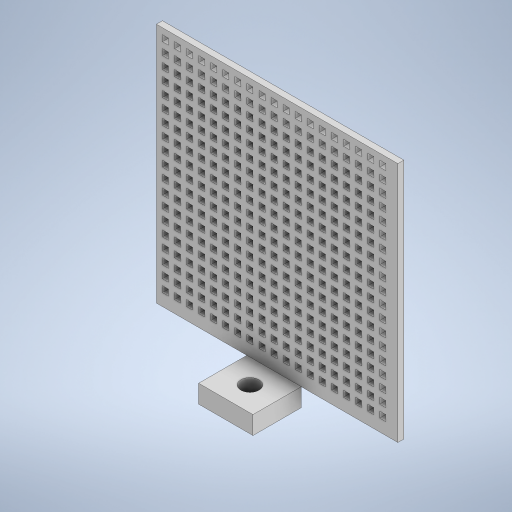
# Autodesk Inventor part: grating20
Saved by Autodesk Inventor 2023 (Build 270158000, 158)
## iProperties
Created: 2022-05-17
Part Number: grating20
Material: Generisch
Document SubType Name: Modeling
Designer: Tim Stechel
Density: 1 g/cm^3
Appearance: Vorgabe
Author: Tim Stechel
Autodesk Inventor part; units mm, degrees
ref_plane "YZ Plane" through (0, 0, 0) normal (1, 0, 0) x (0, 1, 0)
ref_plane "XZ Plane" through (0, 0, 0) normal (0, 1, 0) x (-1, 0, 0)
ref_plane "XY Plane" through (0, 0, 0) normal (0, 0, 1) x (1, 0, 0)
sketch "Skizze1" plane through (0, 0, 0) normal (0, 0, 1) x (1, 0, 0)
  line L0 (-20, 20) -> (20, 20)
  line L1 (20, 20) -> (20, -20)
  line L2 (20, -20) -> (-20, -20)
  line L3 (-20, -20) -> (-20, 20)
  line L4 (0, 2.5115) -> (0, -3.4037)
  line L5 (3.1615, 0) -> (-2.0751, 0)
  line L6 (-20, 20) -> (-19.6762, 20)
  line L7 (-20, 20) -> (-19.6762, 20)
  line L8 (-20, 20) -> (-19, 20)
  line L9 (-19, 20) -> (-18, 20)
  line L10 (-20, 20) -> (-19, 20)
  line L11 (-20, 20) -> (-19, 20)
  line L12 (-20, 20) -> (-19, 20)
  line L13 (-19, 20) -> (-18, 20)
  line L14 (-19, 20) -> (-19, -20)
  line L15 (-18, 20) -> (-18, -20)
  line L16 (-18, 20) -> (-17, 20)
  line L17 (-17, 20) -> (-17, -20)
  line L18 (-18, 20) -> (-18, -20)
  line L19 (-17, 20) -> (-16, 20)
  line L20 (-16, 20) -> (-16, -20)
  line L21 (-17, 20) -> (-17, -20)
  line L22 (-16, 20) -> (-15, 20)
  line L23 (-15, 20) -> (-15, -20)
  line L24 (-16, 20) -> (-16, -20)
  line L25 (-15, 20) -> (-14, 20)
  line L26 (-14, 20) -> (-14, -20)
  line L27 (-15, 20) -> (-15, -20)
  line L28 (-14, 20) -> (-13, 20)
  line L29 (-13, 20) -> (-13, -20)
  line L30 (-14, 20) -> (-14, -20)
  line L31 (-13, 20) -> (-12, 20)
  line L32 (-12, 20) -> (-12, -20)
  line L33 (-13, 20) -> (-13, -20)
  line L34 (-12, 20) -> (-11, 20)
  line L35 (-11, 20) -> (-11, -20)
  line L36 (-12, 20) -> (-12, -20)
  line L37 (-11, 20) -> (-10, 20)
  line L38 (-10, 20) -> (-10, -20)
  line L39 (-11, 20) -> (-11, -20)
  line L40 (-10, 20) -> (-9, 20)
  line L41 (-9, 20) -> (-9, -20)
  line L42 (-10, 20) -> (-10, -20)
  line L43 (-9, 20) -> (-8, 20)
  line L44 (-8, 20) -> (-8, -20)
  line L45 (-9, 20) -> (-9, -20)
  line L46 (-8, 20) -> (-7, 20)
  line L47 (-7, 20) -> (-7, -20)
  line L48 (-8, 20) -> (-8, -20)
  line L49 (-7, 20) -> (-6, 20)
  line L50 (-6, 20) -> (-6, -20)
  line L51 (-7, 20) -> (-7, -20)
  line L52 (-6, 20) -> (-5, 20)
  line L53 (-5, 20) -> (-5, -20)
  line L54 (-6, 20) -> (-6, -20)
  line L55 (-5, 20) -> (-4, 20)
  line L56 (-4, 20) -> (-4, -20)
  line L57 (-5, 20) -> (-5, -20)
  line L58 (-4, 20) -> (-3, 20)
  line L59 (-3, 20) -> (-3, -20)
  line L60 (-4, 20) -> (-4, -20)
  line L61 (-3, 20) -> (-2, 20)
  line L62 (-2, 20) -> (-2, -20)
  line L63 (-3, 20) -> (-3, -20)
  line L64 (-2, 20) -> (-1, 20)
  line L65 (-1, 20) -> (-1, -20)
  line L66 (-2, 20) -> (-2, -20)
  line L67 (-1, 20) -> (0, 20)
  line L68 (0, 20) -> (0, -20)
  line L69 (-1, 20) -> (-1, -20)
  line L70 (0, 20) -> (1, 20)
  line L71 (1, 20) -> (1, -20)
  line L72 (0, 20) -> (0, -20)
  line L73 (1, 20) -> (2, 20)
  line L74 (2, 20) -> (2, -20)
  line L75 (1, 20) -> (1, -20)
  line L76 (2, 20) -> (3, 20)
  line L77 (3, 20) -> (3, -20)
  line L78 (2, 20) -> (2, -20)
  line L79 (3, 20) -> (4, 20)
  line L80 (4, 20) -> (4, -20)
  line L81 (3, 20) -> (3, -20)
  line L82 (4, 20) -> (5, 20)
  line L83 (5, 20) -> (5, -20)
  line L84 (4, 20) -> (4, -20)
  line L85 (5, 20) -> (6, 20)
  line L86 (6, 20) -> (6, -20)
  line L87 (5, 20) -> (5, -20)
  line L88 (6, 20) -> (7, 20)
  line L89 (7, 20) -> (7, -20)
  line L90 (6, 20) -> (6, -20)
  line L91 (7, 20) -> (8, 20)
  line L92 (8, 20) -> (8, -20)
  line L93 (7, 20) -> (7, -20)
  line L94 (8, 20) -> (9, 20)
  line L95 (9, 20) -> (9, -20)
  line L96 (8, 20) -> (8, -20)
  line L97 (9, 20) -> (10, 20)
  line L98 (10, 20) -> (10, -20)
  line L99 (9, 20) -> (9, -20)
  line L100 (10, 20) -> (11, 20)
  line L101 (11, 20) -> (11, -20)
  line L102 (10, 20) -> (10, -20)
  line L103 (11, 20) -> (12, 20)
  line L104 (12, 20) -> (12, -20)
  line L105 (11, 20) -> (11, -20)
  line L106 (12, 20) -> (13, 20)
  line L107 (13, 20) -> (13, -20)
  line L108 (12, 20) -> (12, -20)
  line L109 (13, 20) -> (14, 20)
  line L110 (14, 20) -> (14, -20)
  line L111 (13, 20) -> (13, -20)
  line L112 (14, 20) -> (15, 20)
  line L113 (15, 20) -> (15, -20)
  line L114 (14, 20) -> (14, -20)
  line L115 (15, 20) -> (16, 20)
  line L116 (16, 20) -> (16, -20)
  line L117 (15, 20) -> (15, -20)
  line L118 (16, 20) -> (17, 20)
  line L119 (17, 20) -> (17, -20)
  line L120 (16, 20) -> (16, -20)
  line L121 (17, 20) -> (18, 20)
  line L122 (18, 20) -> (18, -20)
  line L123 (17, 20) -> (17, -20)
  line L124 (18, 20) -> (19, 20)
  line L125 (19, 20) -> (19, -20)
  line L126 (18, 20) -> (18, -20)
  line L127 (-20, -20) -> (-20, -19)
  line L128 (-20, -19) -> (-20, -18)
  line L129 (-20, -18) -> (20, -18)
  line L130 (-20, -19) -> (20, -19)
  line L131 (-20, -18) -> (20, -18)
  line L132 (-20, -17) -> (20, -17)
  line L133 (-20, -17) -> (20, -17)
  line L134 (-20, -16) -> (20, -16)
  line L135 (-20, -16) -> (20, -16)
  line L136 (-20, -15) -> (20, -15)
  line L137 (-20, -15) -> (20, -15)
  line L138 (-20, -14) -> (20, -14)
  line L139 (-20, -14) -> (20, -14)
  line L140 (-20, -13) -> (20, -13)
  line L141 (-20, -13) -> (20, -13)
  line L142 (-20, -12) -> (20, -12)
  line L143 (-20, -12) -> (20, -12)
  line L144 (-20, -11) -> (20, -11)
  line L145 (-20, -11) -> (20, -11)
  line L146 (-20, -10) -> (20, -10)
  line L147 (-20, -10) -> (20, -10)
  line L148 (-20, -9) -> (20, -9)
  line L149 (-20, -9) -> (20, -9)
  line L150 (-20, -8) -> (20, -8)
  line L151 (-20, -8) -> (20, -8)
  line L152 (-20, -7) -> (20, -7)
  line L153 (-20, -7) -> (20, -7)
  line L154 (-20, -6) -> (20, -6)
  line L155 (-20, -6) -> (20, -6)
  line L156 (-20, -5) -> (20, -5)
  line L157 (-20, -5) -> (20, -5)
  line L158 (-20, -4) -> (20, -4)
  line L159 (-20, -4) -> (20, -4)
  line L160 (-20, -3) -> (20, -3)
  line L161 (-20, -3) -> (20, -3)
  line L162 (-20, -2) -> (20, -2)
  line L163 (-20, -2) -> (20, -2)
  line L164 (-20, -1) -> (20, -1)
  line L165 (-20, -1) -> (20, -1)
  line L166 (-20, 0) -> (20, 0)
  line L167 (-20, 0) -> (20, 0)
  line L168 (-20, 1) -> (20, 1)
  line L169 (-20, 1) -> (20, 1)
  line L170 (-20, 2) -> (20, 2)
  line L171 (-20, 2) -> (20, 2)
  line L172 (-20, 3) -> (20, 3)
  line L173 (-20, 3) -> (20, 3)
  line L174 (-20, 4) -> (20, 4)
  line L175 (-20, 4) -> (20, 4)
  line L176 (-20, 5) -> (20, 5)
  line L177 (-20, 5) -> (20, 5)
  line L178 (-20, 6) -> (20, 6)
  line L179 (-20, 6) -> (20, 6)
  line L180 (-20, 7) -> (20, 7)
  line L181 (-20, 7) -> (20, 7)
  line L182 (-20, 8) -> (20, 8)
  line L183 (-20, 8) -> (20, 8)
  line L184 (-20, 9) -> (20, 9)
  line L185 (-20, 9) -> (20, 9)
  line L186 (-20, 10) -> (20, 10)
  line L187 (-20, 10) -> (20, 10)
  line L188 (-20, 11) -> (20, 11)
  line L189 (-20, 11) -> (20, 11)
  line L190 (-20, 12) -> (20, 12)
  line L191 (-20, 12) -> (20, 12)
  line L192 (-20, 13) -> (20, 13)
  line L193 (-20, 13) -> (20, 13)
  line L194 (-20, 14) -> (20, 14)
  line L195 (-20, 14) -> (20, 14)
  line L196 (-20, 15) -> (20, 15)
  line L197 (-20, 15) -> (20, 15)
  line L198 (-20, 16) -> (20, 16)
  line L199 (-20, 16) -> (20, 16)
  line L200 (-20, 17) -> (20, 17)
  line L201 (-20, 17) -> (20, 17)
  line L202 (-20, 18) -> (20, 18)
  line L203 (-20, 18) -> (20, 18)
  line L204 (-20, 19) -> (20, 19)
  point P0 (0, 0)
  point P1 (0, 0)
  point P2 (0, 0)
  point P3 (-20, 0)
  point P4 (20, 0)
  point P5 (0, 0)
  point P6 (0, 0)
  point P7 (0, 20)
  point P8 (0, 0)
  point P9 (0, 0)
  dimension "d1" = 40
  dimension "d2" = 40
  dimension "int" = 1
  dimension "d9" = 1
  dimension "d10" = 40
  dimension "d11" = 40
  dimension "d21" = 1
  dimension "d22" = 1
  dimension "d23" = 40
  dimension "d24" = 40
  dimension "d27" = 1
  constraints: 406 end point, 6 coincident, 5 point on line, 3 horizontal, 3 vertical, 2 midpoint, 1 collinear, 1 parallel, 235 other
  measures "d1" distance of L3.end L1.start
  measures "d2" distance of L1.start L1.end
  measures "int" distance of L3.end L8.end
  measures "d9" distance of L8.end L9.end
  measures "d10" distance of L8.end L14.end
  measures "d11" distance of L9.end L15.end
  measures "d21" distance of L3.start L127.end
  measures "d22" distance of L127.end L128.end
  measures "d23" distance of L128.end L129.end
  measures "d24" distance of L127.end L130.end
  measures "d27" distance of L127.end L131.start
extrude "Extrusion1" add sketch "Skizze1" along normal blind 1 contours L0 L14 L204 L3 | L204 L14 L202 L3 | L202 L14 L200 L3 | L0 L17 L204 L15 | L200 L14 L198 L3 | L204 L17 L202 L15 | L198 L14 L196 L3 | L202 L17 L200 L15 | L0 L23 L204 L20 | L196 L14 L194 L3 | L200 L17 L198 L15 | L204 L23 L202 L20 | L194 L14 L192 L3 | L198 L17 L196 L15 | L202 L23 L200 L20 | L0 L29 L204 L26 | L192 L14 L190 L3 | L196 L17 L194 L15 | L200 L23 L198 L20 | L204 L29 L202 L26 | L190 L14 L188 L3 | L194 L17 L192 L15 | L198 L23 L196 L20 | L202 L29 L200 L26 | L0 L35 L204 L32 | L188 L14 L186 L3 | L192 L17 L190 L15 | L196 L23 L194 L20 | L200 L29 L198 L26 | L204 L35 L202 L32 | L186 L14 L184 L3 | L190 L17 L188 L15 | L194 L23 L192 L20 | L198 L29 L196 L26 | L202 L35 L200 L32 | L0 L41 L204 L38 | L184 L14 L182 L3 | L188 L17 L186 L15 | L192 L23 L190 L20 | L196 L29 L194 L26 | L200 L35 L198 L32 | L204 L41 L202 L38 | L182 L14 L180 L3 | L186 L17 L184 L15 | L190 L23 L188 L20 | L194 L29 L192 L26 | L198 L35 L196 L32 | L202 L41 L200 L38 | L0 L47 L204 L44 | L180 L14 L178 L3 | L184 L17 L182 L15 | L188 L23 L186 L20 | L192 L29 L190 L26 | L196 L35 L194 L32 | L200 L41 L198 L38 | L204 L47 L202 L44 | L178 L14 L176 L3 | L182 L17 L180 L15 | L186 L23 L184 L20 | L190 L29 L188 L26 | L194 L35 L192 L32 | L198 L41 L196 L38 | L202 L47 L200 L44 | L0 L53 L204 L50 | L176 L14 L174 L3 | L180 L17 L178 L15 | L184 L23 L182 L20 | L188 L29 L186 L26 | L192 L35 L190 L32 | L196 L41 L194 L38 | L200 L47 L198 L44 | L204 L53 L202 L50 | L174 L14 L172 L3 | L178 L17 L176 L15 | L182 L23 L180 L20 | L186 L29 L184 L26 | L190 L35 L188 L32 | L194 L41 L192 L38 | L198 L47 L196 L44 | L202 L53 L200 L50 | L0 L59 L204 L56 | L172 L14 L170 L3 | L176 L17 L174 L15 | L180 L23 L178 L20 | L184 L29 L182 L26 | L188 L35 L186 L32 | L192 L41 L190 L38 | L196 L47 L194 L44 | L200 L53 L198 L50 | L204 L59 L202 L56 | L170 L14 L168 L3 | L174 L17 L172 L15 | L178 L23 L176 L20 | L182 L29 L180 L26 | L186 L35 L184 L32 | L190 L41 L188 L38 | L194 L47 L192 L44 | L198 L53 L196 L50 | L202 L59 L200 L56 | L0 L65 L204 L62 | L168 L14 L166 L3 | L172 L17 L170 L15 | L176 L23 L174 L20 | L180 L29 L178 L26 | L184 L35 L182 L32 | L188 L41 L186 L38 | L192 L47 L190 L44 | L196 L53 L194 L50 | L200 L59 L198 L56 | L204 L65 L202 L62 | L166 L14 L164 L3 | L170 L17 L168 L15 | L174 L23 L172 L20 | L178 L29 L176 L26 | L182 L35 L180 L32 | L186 L41 L184 L38 | L190 L47 L188 L44 | L194 L53 L192 L50 | L198 L59 L196 L56 | L202 L65 L200 L62 | L0 L71 L204 L68 | L164 L14 L162 L3 | L168 L17 L166 L15 | L172 L23 L170 L20 | L176 L29 L174 L26 | L180 L35 L178 L32 | L184 L41 L182 L38 | L188 L47 L186 L44 | L192 L53 L190 L50 | L196 L59 L194 L56 | L200 L65 L198 L62 | L204 L71 L202 L68 | L162 L14 L160 L3 | L166 L17 L164 L15 | L170 L23 L168 L20 | L174 L29 L172 L26 | L178 L35 L176 L32 | L182 L41 L180 L38 | L186 L47 L184 L44 | L190 L53 L188 L50 | L194 L59 L192 L56 | L198 L65 L196 L62 | L202 L71 L200 L68 | L0 L77 L204 L74 | L160 L14 L158 L3 | L164 L17 L162 L15 | L168 L23 L166 L20 | L172 L29 L170 L26 | L176 L35 L174 L32 | L180 L41 L178 L38 | L184 L47 L182 L44 | L188 L53 L186 L50 | L192 L59 L190 L56 | L196 L65 L194 L62 | L200 L71 L198 L68 | L204 L77 L202 L74 | L158 L14 L156 L3 | L162 L17 L160 L15 | L166 L23 L164 L20 | L170 L29 L168 L26 | L174 L35 L172 L32 | L178 L41 L176 L38 | L182 L47 L180 L44 | L186 L53 L184 L50 | L190 L59 L188 L56 | L194 L65 L192 L62 | L198 L71 L196 L68 | L202 L77 L200 L74 | L0 L83 L204 L80 | L156 L14 L154 L3 | L160 L17 L158 L15 | L164 L23 L162 L20 | L168 L29 L166 L26 | L172 L35 L170 L32 | L176 L41 L174 L38 | L180 L47 L178 L44 | L184 L53 L182 L50 | L188 L59 L186 L56 | L192 L65 L190 L62 | L196 L71 L194 L68 | L200 L77 L198 L74 | L204 L83 L202 L80 | L154 L14 L152 L3 | L158 L17 L156 L15 | L162 L23 L160 L20 | L166 L29 L164 L26 | L170 L35 L168 L32 | L174 L41 L172 L38 | L178 L47 L176 L44 | L182 L53 L180 L50 | L186 L59 L184 L56 | L190 L65 L188 L62 | L194 L71 L192 L68 | L198 L77 L196 L74 | L202 L83 L200 L80 | L0 L89 L204 L86 | L152 L14 L150 L3 | L156 L17 L154 L15 | L160 L23 L158 L20 | L164 L29 L162 L26 | L168 L35 L166 L32 | L172 L41 L170 L38 | L176 L47 L174 L44 | L180 L53 L178 L50 | L184 L59 L182 L56 | L188 L65 L186 L62 | L192 L71 L190 L68 | L196 L77 L194 L74 | L200 L83 L198 L80 | L204 L89 L202 L86 | L150 L14 L148 L3 | L154 L17 L152 L15 | L158 L23 L156 L20 | L162 L29 L160 L26 | L166 L35 L164 L32 | L170 L41 L168 L38 | L174 L47 L172 L44 | L178 L53 L176 L50 | L182 L59 L180 L56 | L186 L65 L184 L62 | L190 L71 L188 L68 | L194 L77 L192 L74 | L198 L83 L196 L80 | L202 L89 L200 L86 | L0 L95 L204 L92 | L148 L14 L146 L3 | L152 L17 L150 L15 | L156 L23 L154 L20 | L160 L29 L158 L26 | L164 L35 L162 L32 | L168 L41 L166 L38 | L172 L47 L170 L44 | L176 L53 L174 L50 | L180 L59 L178 L56 | L184 L65 L182 L62 | L188 L71 L186 L68 | L192 L77 L190 L74 | L196 L83 L194 L80 | L200 L89 L198 L86 | L204 L95 L202 L92 | L146 L14 L144 L3 | L150 L17 L148 L15 | L154 L23 L152 L20 | L158 L29 L156 L26 | L162 L35 L160 L32 | L166 L41 L164 L38 | L170 L47 L168 L44 | L174 L53 L172 L50 | L178 L59 L176 L56 | L182 L65 L180 L62 | L186 L71 L184 L68 | L190 L77 L188 L74 | L194 L83 L192 L80 | L198 L89 L196 L86 | L202 L95 L200 L92 | L0 L101 L204 L98 | L144 L14 L142 L3 | L148 L17 L146 L15 | L152 L23 L150 L20 | L156 L29 L154 L26 | L160 L35 L158 L32 | L164 L41 L162 L38 | L168 L47 L166 L44 | L172 L53 L170 L50 | L176 L59 L174 L56 | L180 L65 L178 L62 | L184 L71 L182 L68 | L188 L77 L186 L74 | L192 L83 L190 L80 | L196 L89 L194 L86 | L200 L95 L198 L92 | L204 L101 L202 L98 | L142 L14 L140 L3 | L146 L17 L144 L15 | L150 L23 L148 L20 | L154 L29 L152 L26 | L158 L35 L156 L32 | L162 L41 L160 L38 | L166 L47 L164 L44 | L170 L53 L168 L50 | L174 L59 L172 L56 | L178 L65 L176 L62 | L182 L71 L180 L68 | L186 L77 L184 L74 | L190 L83 L188 L80 | L194 L89 L192 L86 | L198 L95 L196 L92 | L202 L101 L200 L98 | L0 L107 L204 L104 | L140 L14 L138 L3 | L144 L17 L142 L15 | L148 L23 L146 L20 | L152 L29 L150 L26 | L156 L35 L154 L32 | L160 L41 L158 L38 | L164 L47 L162 L44 | L168 L53 L166 L50 | L172 L59 L170 L56 | L176 L65 L174 L62 | L180 L71 L178 L68 | L184 L77 L182 L74 | L188 L83 L186 L80 | L192 L89 L190 L86 | L196 L95 L194 L92 | L200 L101 L198 L98 | L204 L107 L202 L104 | L138 L14 L136 L3 | L142 L17 L140 L15 | L146 L23 L144 L20 | L150 L29 L148 L26 | L154 L35 L152 L32 | L158 L41 L156 L38 | L162 L47 L160 L44 | L166 L53 L164 L50 | L170 L59 L168 L56 | L174 L65 L172 L62 | L178 L71 L176 L68 | L182 L77 L180 L74 | L186 L83 L184 L80 | L190 L89 L188 L86 | L194 L95 L192 L92 | L198 L101 L196 L98 | L202 L107 L200 L104 | L0 L113 L204 L110 | L136 L14 L134 L3 | L140 L17 L138 L15 | L144 L23 L142 L20 | L148 L29 L146 L26 | L152 L35 L150 L32 | L156 L41 L154 L38 | L160 L47 L158 L44 | L164 L53 L162 L50 | L168 L59 L166 L56 | L172 L65 L170 L62 | L176 L71 L174 L68 | L180 L77 L178 L74 | L184 L83 L182 L80 | L188 L89 L186 L86 | L192 L95 L190 L92 | L196 L101 L194 L98 | L200 L107 L198 L104 | L204 L113 L202 L110 | L134 L14 L132 L3 | L138 L17 L136 L15 | L142 L23 L140 L20 | L146 L29 L144 L26 | L150 L35 L148 L32 | L154 L41 L152 L38 | L158 L47 L156 L44 | L162 L53 L160 L50 | L166 L59 L164 L56 | L170 L65 L168 L62 | L174 L71 L172 L68 | L178 L77 L176 L74 | L182 L83 L180 L80 | L186 L89 L184 L86 | L190 L95 L188 L92 | L194 L101 L192 L98 | L198 L107 L196 L104 | L202 L113 L200 L110 | L0 L119 L204 L116 | L132 L14 L129 L3 | L136 L17 L134 L15 | L140 L23 L138 L20 | L144 L29 L142 L26 | L148 L35 L146 L32 | L152 L41 L150 L38 | L156 L47 L154 L44 | L160 L53 L158 L50 | L164 L59 L162 L56 | L168 L65 L5 L62 | L172 L71 L170 L4 L68 | L176 L77 L174 L74 | L180 L83 L178 L80 | L184 L89 L182 L86 | L188 L95 L186 L92 | L192 L101 L190 L98 | L196 L107 L194 L104 | L200 L113 L198 L110 | L204 L119 L202 L116 | L129 L14 L130 L3 | L134 L17 L132 L15 | L138 L23 L136 L20 | L142 L29 L140 L26 | L146 L35 L144 L32 | L150 L41 L148 L38 | L154 L47 L152 L44 | L158 L53 L156 L50 | L162 L59 L160 L56 | L5 L65 L164 L62 | L170 L71 L168 L4 | L174 L77 L172 L74 | L178 L83 L176 L80 | L182 L89 L180 L86 | L186 L95 L184 L92 | L190 L101 L188 L98 | L194 L107 L192 L104 | L198 L113 L196 L110 | L202 L119 L200 L116 | L0 L125 L204 L122 | L130 L14 L2 L3 | L132 L17 L129 L15 | L136 L23 L134 L20 | L140 L29 L138 L26 | L144 L35 L142 L32 | L148 L41 L146 L38 | L152 L47 L150 L44 | L156 L53 L154 L50 | L160 L59 L158 L56 | L164 L65 L162 L62 | L168 L71 L5 L4 | L172 L77 L170 L74 | L176 L83 L174 L80 | L180 L89 L178 L86 | L184 L95 L182 L92 | L188 L101 L186 L98 | L192 L107 L190 L104 | L196 L113 L194 L110 | L200 L119 L198 L116 | L204 L125 L202 L122 | L0 L1 L204 L125 | L129 L17 L130 L15 | L134 L23 L132 L20 | L138 L29 L136 L26 | L142 L35 L140 L32 | L146 L41 L144 L38 | L150 L47 L148 L44 | L154 L53 L152 L50 | L158 L59 L156 L56 | L162 L65 L160 L62 | L5 L71 L164 L4 | L170 L77 L168 L74 | L174 L83 L172 L80 | L178 L89 L176 L86 | L182 L95 L180 L92 | L186 L101 L184 L98 | L190 L107 L188 L104 | L194 L113 L192 L110 | L198 L119 L196 L116 | L202 L125 L200 L122 | L204 L1 L202 L125 | L130 L17 L2 L15 | L132 L23 L129 L20 | L136 L29 L134 L26 | L140 L35 L138 L32 | L144 L41 L142 L38 | L148 L47 L146 L44 | L152 L53 L150 L50 | L156 L59 L154 L56 | L160 L65 L158 L62 | L164 L71 L162 L4 | L168 L77 L5 L74 | L172 L83 L170 L80 | L176 L89 L174 L86 | L180 L95 L178 L92 | L184 L101 L182 L98 | L188 L107 L186 L104 | L192 L113 L190 L110 | L196 L119 L194 L116 | L200 L125 L198 L122 | L202 L1 L200 L125 | L129 L23 L130 L20 | L134 L29 L132 L26 | L138 L35 L136 L32 | L142 L41 L140 L38 | L146 L47 L144 L44 | L150 L53 L148 L50 | L154 L59 L152 L56 | L158 L65 L156 L62 | L162 L71 L160 L4 | L5 L77 L164 L74 | L170 L83 L168 L80 | L174 L89 L172 L86 | L178 L95 L176 L92 | L182 L101 L180 L98 | L186 L107 L184 L104 | L190 L113 L188 L110 | L194 L119 L192 L116 | L198 L125 L196 L122 | L200 L1 L198 L125 | L130 L23 L2 L20 | L132 L29 L129 L26 | L136 L35 L134 L32 | L140 L41 L138 L38 | L144 L47 L142 L44 | L148 L53 L146 L50 | L152 L59 L150 L56 | L156 L65 L154 L62 | L160 L71 L158 L68 L4 | L164 L77 L162 L74 | L168 L83 L166 L80 | L172 L89 L170 L86 | L176 L95 L174 L92 | L180 L101 L178 L98 | L184 L107 L182 L104 | L188 L113 L186 L110 | L192 L119 L190 L116 | L196 L125 L194 L122 | L198 L1 L196 L125 | L129 L29 L130 L26 | L134 L35 L132 L32 | L138 L41 L136 L38 | L142 L47 L140 L44 | L146 L53 L144 L50 | L150 L59 L148 L56 | L154 L65 L152 L62 | L158 L71 L156 L68 | L162 L77 L160 L74 | L166 L83 L164 L80 | L170 L89 L168 L86 | L174 L95 L172 L92 | L178 L101 L176 L98 | L182 L107 L180 L104 | L186 L113 L184 L110 | L190 L119 L188 L116 | L194 L125 L192 L122 | L196 L1 L194 L125 | L130 L29 L2 L26 | L132 L35 L129 L32 | L136 L41 L134 L38 | L140 L47 L138 L44 | L144 L53 L142 L50 | L148 L59 L146 L56 | L152 L65 L150 L62 | L156 L71 L154 L68 | L160 L77 L158 L74 | L164 L83 L162 L80 | L168 L89 L166 L86 | L172 L95 L170 L92 | L176 L101 L174 L98 | L180 L107 L178 L104 | L184 L113 L182 L110 | L188 L119 L186 L116 | L192 L125 L190 L122 | L194 L1 L192 L125 | L129 L35 L130 L32 | L134 L41 L132 L38 | L138 L47 L136 L44 | L142 L53 L140 L50 | L146 L59 L144 L56 | L150 L65 L148 L62 | L154 L71 L152 L68 | L158 L77 L156 L74 | L162 L83 L160 L80 | L166 L89 L164 L86 | L170 L95 L168 L92 | L174 L101 L172 L98 | L178 L107 L176 L104 | L182 L113 L180 L110 | L186 L119 L184 L116 | L190 L125 L188 L122 | L192 L1 L190 L125 | L130 L35 L2 L32 | L132 L41 L129 L38 | L136 L47 L134 L44 | L140 L53 L138 L50 | L144 L59 L142 L56 | L148 L65 L146 L62 | L152 L71 L150 L68 | L156 L77 L154 L74 | L160 L83 L158 L80 | L164 L89 L162 L86 | L168 L95 L166 L92 | L172 L101 L170 L98 | L176 L107 L174 L104 | L180 L113 L178 L110 | L184 L119 L182 L116 | L188 L125 L186 L122 | L190 L1 L188 L125 | L129 L41 L130 L38 | L134 L47 L132 L44 | L138 L53 L136 L50 | L142 L59 L140 L56 | L146 L65 L144 L62 | L150 L71 L148 L68 | L154 L77 L152 L74 | L158 L83 L156 L80 | L162 L89 L160 L86 | L166 L95 L164 L92 | L170 L101 L168 L98 | L174 L107 L172 L104 | L178 L113 L176 L110 | L182 L119 L180 L116 | L186 L125 L184 L122 | L188 L1 L186 L125 | L130 L41 L2 L38 | L132 L47 L129 L44 | L136 L53 L134 L50 | L140 L59 L138 L56 | L144 L65 L142 L62 | L148 L71 L146 L68 | L152 L77 L150 L74 | L156 L83 L154 L80 | L160 L89 L158 L86 | L164 L95 L162 L92 | L168 L101 L166 L98 | L172 L107 L170 L104 | L176 L113 L174 L110 | L180 L119 L178 L116 | L184 L125 L182 L122 | L186 L1 L184 L125 | L129 L47 L130 L44 | L134 L53 L132 L50 | L138 L59 L136 L56 | L142 L65 L140 L62 | L146 L71 L144 L68 | L150 L77 L148 L74 | L154 L83 L152 L80 | L158 L89 L156 L86 | L162 L95 L160 L92 | L166 L101 L164 L98 | L170 L107 L168 L104 | L174 L113 L172 L110 | L178 L119 L176 L116 | L182 L125 L180 L122 | L184 L1 L182 L125 | L130 L47 L2 L44 | L132 L53 L129 L50 | L136 L59 L134 L56 | L140 L65 L138 L62 | L144 L71 L142 L68 | L148 L77 L146 L74 | L152 L83 L150 L80 | L156 L89 L154 L86 | L160 L95 L158 L92 | L164 L101 L162 L98 | L168 L107 L166 L104 | L172 L113 L170 L110 | L176 L119 L174 L116 | L180 L125 L178 L122 | L182 L1 L180 L125 | L129 L53 L130 L50 | L134 L59 L132 L56 | L138 L65 L136 L62 | L142 L71 L140 L68 | L146 L77 L144 L74 | L150 L83 L148 L80 | L154 L89 L152 L86 | L158 L95 L156 L92 | L162 L101 L160 L98 | L166 L107 L164 L104 | L170 L113 L168 L110 | L174 L119 L172 L116 | L178 L125 L176 L122 | L180 L1 L178 L125 | L130 L53 L2 L50 | L132 L59 L129 L56 | L136 L65 L134 L62 | L140 L71 L138 L68 | L144 L77 L142 L74 | L148 L83 L146 L80 | L152 L89 L150 L86 | L156 L95 L154 L92 | L160 L101 L158 L98 | L164 L107 L162 L104 | L168 L113 L166 L110 | L172 L119 L170 L116 | L176 L125 L174 L122 | L178 L1 L176 L125 | L129 L59 L130 L56 | L134 L65 L132 L62 | L138 L71 L136 L68 | L142 L77 L140 L74 | L146 L83 L144 L80 | L150 L89 L148 L86 | L154 L95 L152 L92 | L158 L101 L156 L98 | L162 L107 L160 L104 | L166 L113 L164 L110 | L170 L119 L168 L116 | L174 L125 L172 L122 | L176 L1 L174 L125 | L130 L59 L2 L56 | L132 L65 L129 L62 | L136 L71 L134 L68 | L140 L77 L138 L74 | L144 L83 L142 L80 | L148 L89 L146 L86 | L152 L95 L150 L92 | L156 L101 L154 L98 | L160 L107 L158 L104 | L164 L113 L162 L110 | L168 L119 L166 L116 | L172 L125 L170 L122 | L174 L1 L172 L125 | L129 L65 L130 L62 | L134 L71 L132 L68 | L138 L77 L136 L74 | L142 L83 L140 L80 | L146 L89 L144 L86 | L150 L95 L148 L92 | L154 L101 L152 L98 | L158 L107 L156 L104 | L162 L113 L160 L110 | L166 L119 L164 L116 | L170 L125 L168 L122 | L172 L1 L170 L125 | L130 L65 L2 L62 | L132 L71 L129 L68 | L136 L77 L134 L74 | L140 L83 L138 L80 | L144 L89 L142 L86 | L148 L95 L146 L92 | L152 L101 L150 L98 | L156 L107 L154 L104 | L160 L113 L158 L110 | L164 L119 L162 L116 | L168 L125 L166 L122 | L170 L1 L168 L125 | L129 L71 L130 L68 | L134 L77 L132 L74 | L138 L83 L136 L80 | L142 L89 L140 L86 | L146 L95 L144 L92 | L150 L101 L148 L98 | L154 L107 L152 L104 | L158 L113 L156 L110 | L162 L119 L160 L116 | L166 L125 L164 L122 | L168 L1 L166 L125 | L130 L71 L2 L68 | L132 L77 L129 L74 | L136 L83 L134 L80 | L140 L89 L138 L86 | L144 L95 L142 L92 | L148 L101 L146 L98 | L152 L107 L150 L104 | L156 L113 L154 L110 | L160 L119 L158 L116 | L164 L125 L162 L122 | L166 L1 L164 L125 | L129 L77 L130 L74 | L134 L83 L132 L80 | L138 L89 L136 L86 | L142 L95 L140 L92 | L146 L101 L144 L98 | L150 L107 L148 L104 | L154 L113 L152 L110 | L158 L119 L156 L116 | L162 L125 L160 L122 | L164 L1 L162 L125 | L130 L77 L2 L74 | L132 L83 L129 L80 | L136 L89 L134 L86 | L140 L95 L138 L92 | L144 L101 L142 L98 | L148 L107 L146 L104 | L152 L113 L150 L110 | L156 L119 L154 L116 | L160 L125 L158 L122 | L162 L1 L160 L125 | L129 L83 L130 L80 | L134 L89 L132 L86 | L138 L95 L136 L92 | L142 L101 L140 L98 | L146 L107 L144 L104 | L150 L113 L148 L110 | L154 L119 L152 L116 | L158 L125 L156 L122 | L160 L1 L158 L125 | L130 L83 L2 L80 | L132 L89 L129 L86 | L136 L95 L134 L92 | L140 L101 L138 L98 | L144 L107 L142 L104 | L148 L113 L146 L110 | L152 L119 L150 L116 | L156 L125 L154 L122 | L158 L1 L156 L125 | L129 L89 L130 L86 | L134 L95 L132 L92 | L138 L101 L136 L98 | L142 L107 L140 L104 | L146 L113 L144 L110 | L150 L119 L148 L116 | L154 L125 L152 L122 | L156 L1 L154 L125 | L130 L89 L2 L86 | L132 L95 L129 L92 | L136 L101 L134 L98 | L140 L107 L138 L104 | L144 L113 L142 L110 | L148 L119 L146 L116 | L152 L125 L150 L122 | L154 L1 L152 L125 | L129 L95 L130 L92 | L134 L101 L132 L98 | L138 L107 L136 L104 | L142 L113 L140 L110 | L146 L119 L144 L116 | L150 L125 L148 L122 | L152 L1 L150 L125 | L130 L95 L2 L92 | L132 L101 L129 L98 | L136 L107 L134 L104 | L140 L113 L138 L110 | L144 L119 L142 L116 | L148 L125 L146 L122 | L150 L1 L148 L125 | L129 L101 L130 L98 | L134 L107 L132 L104 | L138 L113 L136 L110 | L142 L119 L140 L116 | L146 L125 L144 L122 | L148 L1 L146 L125 | L130 L101 L2 L98 | L132 L107 L129 L104 | L136 L113 L134 L110 | L140 L119 L138 L116 | L144 L125 L142 L122 | L146 L1 L144 L125 | L129 L107 L130 L104 | L134 L113 L132 L110 | L138 L119 L136 L116 | L142 L125 L140 L122 | L144 L1 L142 L125 | L130 L107 L2 L104 | L132 L113 L129 L110 | L136 L119 L134 L116 | L140 L125 L138 L122 | L142 L1 L140 L125 | L129 L113 L130 L110 | L134 L119 L132 L116 | L138 L125 L136 L122 | L140 L1 L138 L125 | L130 L113 L2 L110 | L132 L119 L129 L116 | L136 L125 L134 L122 | L138 L1 L136 L125 | L129 L119 L130 L116 | L134 L125 L132 L122 | L136 L1 L134 L125 | L130 L119 L2 L116 | L132 L125 L129 L122 | L134 L1 L132 L125 | L129 L125 L130 L122 | L132 L1 L129 L125 | L130 L125 L2 L122 | L129 L1 L130 L125 | L130 L1 L2 L125
sketch "Skizze2" plane through (0, 0, 0) normal (0, 0, 1) x (1, 0, 0)
  line L0 (-20, -20) -> (-19, -20) projected
  line L1 (-20, -20) -> (-20, -19)
  line L2 (-20, 20) -> (-20, -20) projected
  line L3 (-20, -19) -> (-20, -18)
  line L4 (-20, -18) -> (20, -18)
  line L5 (20, -20) -> (20, 20) projected
  line L6 (-20, -19) -> (20, -19)
  line L7 (-20, -20) -> (20, -20)
  line L8 (-20, -18) -> (20, -18)
  line L9 (-20, -18) -> (-20, -17)
  line L10 (-20, -17) -> (20, -17)
  line L11 (-20, -17) -> (20, -17)
  line L12 (-20, -17) -> (-20, -16)
  line L13 (-20, -16) -> (20, -16)
  line L14 (-20, -16) -> (20, -16)
  line L15 (-20, -16) -> (-20, -15)
  line L16 (-20, -15) -> (20, -15)
  line L17 (-20, -15) -> (20, -15)
  line L18 (-20, -15) -> (-20, -14)
  line L19 (-20, -14) -> (20, -14)
  line L20 (-20, -14) -> (20, -14)
  line L21 (-20, -14) -> (-20, -13)
  line L22 (-20, -13) -> (20, -13)
  line L23 (-20, -13) -> (20, -13)
  line L24 (-20, -13) -> (-20, -12)
  line L25 (-20, -12) -> (20, -12)
  line L26 (-20, -12) -> (20, -12)
  line L27 (-20, -12) -> (-20, -11)
  line L28 (-20, -11) -> (20, -11)
  line L29 (-20, -11) -> (20, -11)
  line L30 (-20, -11) -> (-20, -10)
  line L31 (-20, -10) -> (20, -10)
  line L32 (-20, -10) -> (20, -10)
  line L33 (-20, -10) -> (-20, -9)
  line L34 (-20, -9) -> (20, -9)
  line L35 (-20, -9) -> (20, -9)
  line L36 (-20, -9) -> (-20, -8)
  line L37 (-20, -8) -> (20, -8)
  line L38 (-20, -8) -> (20, -8)
  line L39 (-20, -8) -> (-20, -7)
  line L40 (-20, -7) -> (20, -7)
  line L41 (-20, -7) -> (20, -7)
  line L42 (-20, -7) -> (-20, -6)
  line L43 (-20, -6) -> (20, -6)
  line L44 (-20, -6) -> (20, -6)
  line L45 (-20, -6) -> (-20, -5)
  line L46 (-20, -5) -> (20, -5)
  line L47 (-20, -5) -> (20, -5)
  line L48 (-20, -5) -> (-20, -4)
  line L49 (-20, -4) -> (20, -4)
  line L50 (-20, -4) -> (20, -4)
  line L51 (-20, -4) -> (-20, -3)
  line L52 (-20, -3) -> (20, -3)
  line L53 (-20, -3) -> (20, -3)
  line L54 (-20, -3) -> (-20, -2)
  line L55 (-20, -2) -> (20, -2)
  line L56 (-20, -2) -> (20, -2)
  line L57 (-20, -2) -> (-20, -1)
  line L58 (-20, -1) -> (20, -1)
  line L59 (-20, -1) -> (20, -1)
  line L60 (-20, -1) -> (-20, 0)
  line L61 (-20, 0) -> (20, 0)
  line L62 (-20, 0) -> (20, 0)
  line L63 (-20, 0) -> (-20, 1)
  line L64 (-20, 1) -> (20, 1)
  line L65 (-20, 1) -> (20, 1)
  line L66 (-20, 1) -> (-20, 2)
  line L67 (-20, 2) -> (20, 2)
  line L68 (-20, 2) -> (20, 2)
  line L69 (-20, 2) -> (-20, 3)
  line L70 (-20, 3) -> (20, 3)
  line L71 (-20, 3) -> (20, 3)
  line L72 (-20, 3) -> (-20, 4)
  line L73 (-20, 4) -> (20, 4)
  line L74 (-20, 4) -> (20, 4)
  line L75 (-20, 4) -> (-20, 5)
  line L76 (-20, 5) -> (20, 5)
  line L77 (-20, 5) -> (20, 5)
  line L78 (-20, 5) -> (-20, 6)
  line L79 (-20, 6) -> (20, 6)
  line L80 (-20, 6) -> (20, 6)
  line L81 (-20, 6) -> (-20, 7)
  line L82 (-20, 7) -> (20, 7)
  line L83 (-20, 7) -> (20, 7)
  line L84 (-20, 7) -> (-20, 8)
  line L85 (-20, 8) -> (20, 8)
  line L86 (-20, 8) -> (20, 8)
  line L87 (-20, 8) -> (-20, 9)
  line L88 (-20, 9) -> (20, 9)
  line L89 (-20, 9) -> (20, 9)
  line L90 (-20, 9) -> (-20, 10)
  line L91 (-20, 10) -> (20, 10)
  line L92 (-20, 10) -> (20, 10)
  line L93 (-20, 10) -> (-20, 11)
  line L94 (-20, 11) -> (20, 11)
  line L95 (-20, 11) -> (20, 11)
  line L96 (-20, 11) -> (-20, 12)
  line L97 (-20, 12) -> (20, 12)
  line L98 (-20, 12) -> (20, 12)
  line L99 (-20, 12) -> (-20, 13)
  line L100 (-20, 13) -> (20, 13)
  line L101 (-20, 13) -> (20, 13)
  line L102 (-20, 13) -> (-20, 14)
  line L103 (-20, 14) -> (20, 14)
  line L104 (-20, 14) -> (20, 14)
  line L105 (-20, 14) -> (-20, 15)
  line L106 (-20, 15) -> (20, 15)
  line L107 (-20, 15) -> (20, 15)
  line L108 (-20, 15) -> (-20, 16)
  line L109 (-20, 16) -> (20, 16)
  line L110 (-20, 16) -> (20, 16)
  line L111 (-20, 16) -> (-20, 17)
  line L112 (-20, 17) -> (20, 17)
  line L113 (-20, 17) -> (20, 17)
  line L114 (-20, 17) -> (-20, 18)
  line L115 (-20, 18) -> (20, 18)
  line L116 (-20, 18) -> (20, 18)
  line L117 (-20, 18) -> (-20, 19)
  line L118 (-20, 19) -> (20, 19)
  line L119 (-20, 20) -> (20, 20)
  line L120 (-6, 20) -> (-6, -20) projected
  point P0 (0, 0)
  point P1 (20, -4)
  point P2 (20, -3)
  point P3 (20, -2)
  point P4 (20, -1)
  point P5 (20, 0)
  point P6 (20, 1)
  point P7 (20, 2)
  point P8 (20, 3)
  point P9 (20, 4)
  point P10 (20, 5)
  point P11 (20, 6)
  point P12 (20, 7)
  point P13 (20, 8)
  dimension "int1" = 1
  dimension "d33" = 1
  dimension "d37" = 1
  dimension "d42" = 40
  constraints: 234 end point, 148 vertical alignment, 74 parallel, 37 collinear, 3 horizontal, 1 perpendicular, 6 other
  measures "int1" distance of L0.start L1.end
  measures "d33" distance of L1.end L3.end
  measures "d37" distance of L1.end L8.start
  measures "d42" distance of L119.start L119.end
extrude "Extrusion2" add sketch "Skizze2" along normal blind 1 contours L1 L6 L120 L7 L0 | L2 L4 L120 L6 | L120 L6 L5 L7 | L120 L4 L5 L6 | L2 L13 L120 L10 | L120 L13 L5 L10 | L2 L19 L120 L16 | L120 L19 L5 L16 | L2 L25 L120 L22 | L120 L25 L5 L22 | L2 L31 L120 L28 | L120 L31 L5 L28 | L2 L37 L120 L34 | L120 L37 L5 L34 | L2 L43 L120 L40 | L120 L43 L5 L40 | L2 L49 L120 L46 | L120 L49 L5 L46 | L2 L55 L120 L52 | L120 L55 L5 L52 | L2 L61 L120 L58 | L120 L61 L5 L58 | L2 L67 L120 L64 | L120 L67 L5 L64 | L2 L73 L120 L70 | L120 L73 L5 L70 | L2 L79 L120 L76 | L120 L79 L5 L76 | L2 L85 L120 L82 | L120 L85 L5 L82 | L2 L91 L120 L88 | L120 L91 L5 L88 | L2 L97 L120 L94 | L120 L97 L5 L94 | L2 L103 L120 L100 | L120 L103 L5 L100 | L2 L109 L120 L106 | L120 L109 L5 L106 | L2 L115 L120 L112 | L120 L115 L5 L112 | L2 L119 L120 L118 | L120 L119 L5 L118
sketch "Skizze3" plane through (0, 0, 1) normal (0, 0, 1) x (1, 0, 0)
  line L0 (-4, -18) -> (-5, -18) projected
  line L1 (-5, -18) -> (4, -18)
  line L2 (4, -18) -> (4, -23)
  line L3 (4, -23) -> (-5, -23)
  line L4 (-5, -23) -> (-5, -18)
  line L5 (-20, -20) -> (20, -20) projected
  line L6 (-5, -20) -> (4, -20)
  point P0 (0, 0)
  dimension "d45" = 5
  dimension "d46" = 9
  constraints: 10 end point, 4 point on line, 2 parallel, 1 horizontal, 1 perpendicular
  measures "d45" distance of L1.end L2.end
  measures "d46" distance of L2.end L3.end
extrude "Extrusion3" add sketch "Skizze3" along normal blind 8 contours L5 L2 L3 L4
sketch "Skizze4" plane through (-5, -20, 1) normal (0, 1, 0) x (1, 0, 0)
  line L0 (9, -8) -> (0, -8) projected
  line L1 (9, 1) -> (9, 0) projected
  line L2 (0, -8) -> (9, 0)
  line L3 (9, 0) -> (0, 0)
  line L4 (0, 0) -> (9, -8)
  circle A0 centre (4.5, -4) radius 1.5
  point P0 (5, 1)
  dimension "d49" = 3
  constraints: 6 end point, 1 centre point, 1 midpoint, 1 perpendicular
  measures "d49" diameter of A0
hole "Bohrung1" at (-0.5, -20, 5) direction (0, -1, 0) diameter 3 end through all
equation "\"d2\" = d1"
equation "\"int\" = 0.025 * d1"
equation "\"d9\" = int"
equation "\"d10\" = d1"
equation "\"d11\" = d1"
equation "\"d21\" = int"
equation "\"d22\" = int"
equation "\"d23\" = d1"
equation "\"d24\" = d1"
equation "\"d33\" = int1"
